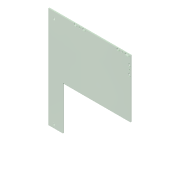
# Autodesk Inventor part: EE PSU TOP
Saved by Autodesk Inventor 2017 (Build 210142000, 142)
## iProperties
Created: 2016-07-27
Part Number: EE PSU TOP
Material: Polycarbonate, Green
Document SubType Name: Modeling
Designer: User
Density: 1.2 g/cm^3
Appearance: Polycarbonate - Clear(2)
Author: User
Autodesk Inventor part; units mm, degrees
ref_plane "YZ Plane" through (0, 0, 0) normal (1, 0, 0) x (0, 1, 0)
ref_plane "XZ Plane" through (0, 0, 0) normal (0, 1, 0) x (-1, 0, 0)
ref_plane "XY Plane" through (0, 0, 0) normal (0, 0, 1) x (1, 0, 0)
sketch "Sketch1" plane through (0, 0, 0) normal (0, 1, 0) x (-1, 0, 0)
  line L0 (55.2995, 771.1017) -> (53.2995, 771.1017)
  line L1 (53.2995, 771.1017) -> (53.2995, 769.1016)
  line L2 (53.2995, 769.1016) -> (53.2995, 481.7779)
  line L3 (53.2995, 481.7779) -> (65.4836, 481.7779)
  line L4 (65.4836, 481.7779) -> (65.4836, 475.7779)
  line L5 (65.4836, 475.7779) -> (70.4836, 475.7779)
  line L6 (70.4836, 475.7779) -> (70.4836, 481.7779)
  line L7 (70.4836, 481.7779) -> (71.2995, 481.7779)
  line L8 (71.2995, 481.7779) -> (71.2995, 623.7779)
  line L9 (71.2995, 623.7779) -> (225.2995, 623.7779)
  line L10 (225.2995, 623.7779) -> (225.2995, 481.7779)
  line L11 (225.2995, 481.7779) -> (234.2995, 481.7779)
  line L12 (234.2995, 481.7779) -> (234.2995, 476.778)
  line L13 (234.2995, 476.778) -> (262.2995, 476.778)
  line L14 (262.2995, 476.778) -> (262.2995, 771.1017)
  line L15 (262.2995, 771.1017) -> (55.2995, 771.1017)
  line L16 (58.3449, 526.6921) -> (58.1851, 527.078)
  line L17 (58.1851, 527.078) -> (57.9308, 527.4094)
  line L18 (57.9308, 527.4094) -> (57.5994, 527.6636)
  line L19 (57.5994, 527.6636) -> (57.2135, 527.8234)
  line L20 (57.2135, 527.8234) -> (56.7994, 527.878)
  line L21 (56.7994, 527.878) -> (56.3853, 527.8234)
  line L22 (56.3853, 527.8234) -> (55.9994, 527.6636)
  line L23 (55.9994, 527.6636) -> (55.668, 527.4093)
  line L24 (55.668, 527.4093) -> (55.4138, 527.0779)
  line L25 (55.4138, 527.0779) -> (55.254, 526.692)
  line L26 (55.254, 526.692) -> (55.1994, 526.2779)
  line L27 (55.1994, 526.2779) -> (55.254, 525.8638)
  line L28 (55.254, 525.8638) -> (55.4138, 525.4779)
  line L29 (55.4138, 525.4779) -> (55.6681, 525.1465)
  line L30 (55.6681, 525.1465) -> (55.9994, 524.8923)
  line L31 (55.9994, 524.8923) -> (56.3853, 524.7325)
  line L32 (56.3853, 524.7325) -> (56.7992, 524.678)
  line L33 (56.7992, 524.678) -> (57.2135, 524.7325)
  line L34 (57.2135, 524.7325) -> (57.5994, 524.8924)
  line L35 (57.5994, 524.8924) -> (57.9308, 525.1466)
  line L36 (57.9308, 525.1466) -> (58.185, 525.478)
  line L37 (58.185, 525.478) -> (58.3449, 525.864)
  line L38 (58.3449, 525.864) -> (58.3994, 526.2781)
  line L39 (58.3994, 526.2781) -> (58.3449, 526.6921)
  line L40 (185.1711, 767.5014) -> (185.0472, 767.8829)
  line L41 (185.0472, 767.8829) -> (184.8323, 768.2215)
  line L42 (184.8323, 768.2215) -> (184.54, 768.496)
  line L43 (184.54, 768.496) -> (184.1885, 768.6893)
  line L44 (184.1885, 768.6893) -> (183.8, 768.7891)
  line L45 (183.8, 768.7891) -> (183.399, 768.7891)
  line L46 (183.399, 768.7891) -> (183.0105, 768.6893)
  line L47 (183.0105, 768.6893) -> (182.659, 768.4961)
  line L48 (182.659, 768.4961) -> (182.3667, 768.2216)
  line L49 (182.3667, 768.2216) -> (182.1518, 767.8829)
  line L50 (182.1518, 767.8829) -> (182.0278, 767.5015)
  line L51 (182.0278, 767.5015) -> (182.0026, 767.1012)
  line L52 (182.0026, 767.1012) -> (182.0778, 766.7072)
  line L53 (182.0778, 766.7072) -> (182.2485, 766.3443)
  line L54 (182.2485, 766.3443) -> (182.5042, 766.0353)
  line L55 (182.5042, 766.0353) -> (182.8287, 765.7996)
  line L56 (182.8287, 765.7996) -> (183.2016, 765.652)
  line L57 (183.2016, 765.652) -> (183.5994, 765.6017)
  line L58 (183.5994, 765.6017) -> (183.9974, 765.652)
  line L59 (183.9974, 765.652) -> (184.3703, 765.7996)
  line L60 (184.3703, 765.7996) -> (184.6947, 766.0353)
  line L61 (184.6947, 766.0353) -> (184.9504, 766.3444)
  line L62 (184.9504, 766.3444) -> (185.1212, 766.7072)
  line L63 (185.1212, 766.7072) -> (185.1963, 767.1012)
  line L64 (185.1963, 767.1012) -> (185.1711, 767.5014)
  line L65 (76.9712, 767.5015) -> (76.8472, 767.8829)
  line L66 (76.8472, 767.8829) -> (76.6323, 768.2216)
  line L67 (76.6323, 768.2216) -> (76.3399, 768.4961)
  line L68 (76.3399, 768.4961) -> (75.9885, 768.6893)
  line L69 (75.9885, 768.6893) -> (75.6, 768.7891)
  line L70 (75.6, 768.7891) -> (75.199, 768.7891)
  line L71 (75.199, 768.7891) -> (74.8105, 768.6893)
  line L72 (74.8105, 768.6893) -> (74.459, 768.4961)
  line L73 (74.459, 768.4961) -> (74.1667, 768.2216)
  line L74 (74.1667, 768.2216) -> (73.9518, 767.8829)
  line L75 (73.9518, 767.8829) -> (73.8278, 767.5015)
  line L76 (73.8278, 767.5015) -> (73.8027, 767.1012)
  line L77 (73.8027, 767.1012) -> (73.8778, 766.7072)
  line L78 (73.8778, 766.7072) -> (74.0486, 766.3444)
  line L79 (74.0486, 766.3444) -> (74.3042, 766.0353)
  line L80 (74.3042, 766.0353) -> (74.6287, 765.7996)
  line L81 (74.6287, 765.7996) -> (75.0016, 765.652)
  line L82 (75.0016, 765.652) -> (75.3995, 765.6017)
  line L83 (75.3995, 765.6017) -> (75.7974, 765.652)
  line L84 (75.7974, 765.652) -> (76.1703, 765.7996)
  line L85 (76.1703, 765.7996) -> (76.4947, 766.0353)
  line L86 (76.4947, 766.0353) -> (76.7504, 766.3444)
  line L87 (76.7504, 766.3444) -> (76.9212, 766.7072)
  line L88 (76.9212, 766.7072) -> (76.9964, 767.1012)
  line L89 (76.9964, 767.1012) -> (76.9712, 767.5015)
  line L90 (250.722, 522.4271) -> (250.4714, 523.032)
  line L91 (250.4714, 523.032) -> (250.0729, 523.5514)
  line L92 (250.0729, 523.5514) -> (249.5534, 523.9499)
  line L93 (249.5534, 523.9499) -> (248.9485, 524.2005)
  line L94 (248.9485, 524.2005) -> (248.2994, 524.286)
  line L95 (248.2994, 524.286) -> (247.6503, 524.2005)
  line L96 (247.6503, 524.2005) -> (247.0454, 523.95)
  line L97 (247.0454, 523.95) -> (246.526, 523.5514)
  line L98 (246.526, 523.5514) -> (246.1275, 523.0319)
  line L99 (246.1275, 523.0319) -> (245.8769, 522.4271)
  line L100 (245.8769, 522.4271) -> (245.7914, 521.778)
  line L101 (245.7914, 521.778) -> (245.8769, 521.1288)
  line L102 (245.8769, 521.1288) -> (246.1275, 520.524)
  line L103 (246.1275, 520.524) -> (246.526, 520.0045)
  line L104 (246.526, 520.0045) -> (247.0455, 519.606)
  line L105 (247.0455, 519.606) -> (247.6504, 519.3555)
  line L106 (247.6504, 519.3555) -> (248.2995, 519.27)
  line L107 (248.2995, 519.27) -> (248.9486, 519.3554)
  line L108 (248.9486, 519.3554) -> (249.5535, 519.606)
  line L109 (249.5535, 519.606) -> (250.0729, 520.0046)
  line L110 (250.0729, 520.0046) -> (250.4714, 520.524)
  line L111 (250.4714, 520.524) -> (250.722, 521.1289)
  line L112 (250.722, 521.1289) -> (250.8075, 521.7779)
  line L113 (250.8075, 521.7779) -> (250.722, 522.4271)
  line L114 (250.7224, 754.4272) -> (250.4718, 755.0321)
  line L115 (250.4718, 755.0321) -> (250.0733, 755.5515)
  line L116 (250.0733, 755.5515) -> (249.5538, 755.95)
  line L117 (249.5538, 755.95) -> (248.9489, 756.2005)
  line L118 (248.9489, 756.2005) -> (248.2998, 756.286)
  line L119 (248.2998, 756.286) -> (247.6507, 756.2006)
  line L120 (247.6507, 756.2006) -> (247.0458, 755.95)
  line L121 (247.0458, 755.95) -> (246.5264, 755.5515)
  line L122 (246.5264, 755.5515) -> (246.1279, 755.032)
  line L123 (246.1279, 755.032) -> (245.8773, 754.4271)
  line L124 (245.8773, 754.4271) -> (245.7918, 753.778)
  line L125 (245.7918, 753.778) -> (245.8773, 753.1288)
  line L126 (245.8773, 753.1288) -> (246.1279, 752.524)
  line L127 (246.1279, 752.524) -> (246.5264, 752.0045)
  line L128 (246.5264, 752.0045) -> (247.0459, 751.606)
  line L129 (247.0459, 751.606) -> (247.6508, 751.3555)
  line L130 (247.6508, 751.3555) -> (248.2999, 751.27)
  line L131 (248.2999, 751.27) -> (248.949, 751.3555)
  line L132 (248.949, 751.3555) -> (249.5539, 751.606)
  line L133 (249.5539, 751.606) -> (250.0737, 752.0049)
  line L134 (250.0737, 752.0049) -> (250.4719, 752.5239)
  line L135 (250.4719, 752.5239) -> (250.7224, 753.1288)
  line L136 (250.7224, 753.1288) -> (250.8079, 753.7777)
  line L137 (250.8079, 753.7777) -> (250.7224, 754.4272)
  line L138 (82.8995, 769.1016) -> (82.8995, 765.5017)
  line L139 (82.8995, 765.5017) -> (89.0995, 765.5017)
  line L140 (89.0995, 765.5017) -> (89.0995, 769.1016)
  line L141 (89.0995, 769.1016) -> (82.8995, 769.1016)
  line L142 (169.8995, 769.1016) -> (169.8995, 765.5017)
  line L143 (169.8995, 765.5017) -> (176.0995, 765.5017)
  line L144 (176.0995, 765.5017) -> (176.0995, 769.1016)
  line L145 (176.0995, 769.1016) -> (169.8995, 769.1016)
  line L146 (191.0995, 769.1016) -> (191.0995, 765.5017)
  line L147 (191.0995, 765.5017) -> (197.2995, 765.5017)
  line L148 (197.2995, 765.5017) -> (197.2995, 769.1016)
  line L149 (197.2995, 769.1016) -> (191.0995, 769.1016)
  line L150 (55.2995, 518.7672) -> (55.2995, 512.5672)
  line L151 (55.2995, 512.5672) -> (58.8995, 512.5672)
  line L152 (58.8995, 512.5672) -> (58.8995, 518.7672)
  line L153 (58.8995, 518.7672) -> (55.2995, 518.7672)
  line L154 (55.2995, 729.278) -> (55.2995, 723.0779)
  line L155 (55.2995, 723.0779) -> (58.8995, 723.0779)
  line L156 (58.8995, 723.0779) -> (58.8995, 729.278)
  line L157 (58.8995, 729.278) -> (55.2995, 729.278)
  line L158 (58.3568, 737.2044) -> (58.197, 737.5902)
  line L159 (58.197, 737.5902) -> (57.9428, 737.9216)
  line L160 (57.9428, 737.9216) -> (57.6114, 738.1758)
  line L161 (57.6114, 738.1758) -> (57.2255, 738.3357)
  line L162 (57.2255, 738.3357) -> (56.8114, 738.3902)
  line L163 (56.8114, 738.3902) -> (56.3972, 738.3357)
  line L164 (56.3972, 738.3357) -> (56.0113, 738.1758)
  line L165 (56.0113, 738.1758) -> (55.68, 737.9216)
  line L166 (55.68, 737.9216) -> (55.4258, 737.5902)
  line L167 (55.4258, 737.5902) -> (55.2659, 737.2043)
  line L168 (55.2659, 737.2043) -> (55.2114, 736.7902)
  line L169 (55.2114, 736.7902) -> (55.2659, 736.3761)
  line L170 (55.2659, 736.3761) -> (55.4257, 735.9902)
  line L171 (55.4257, 735.9902) -> (55.68, 735.6588)
  line L172 (55.68, 735.6588) -> (56.0114, 735.4046)
  line L173 (56.0114, 735.4046) -> (56.3973, 735.2448)
  line L174 (56.3973, 735.2448) -> (56.8114, 735.1902)
  line L175 (56.8114, 735.1902) -> (57.2255, 735.2447)
  line L176 (57.2255, 735.2447) -> (57.6114, 735.4046)
  line L177 (57.6114, 735.4046) -> (57.9427, 735.6588)
  line L178 (57.9427, 735.6588) -> (58.197, 735.9903)
  line L179 (58.197, 735.9903) -> (58.3568, 736.3762)
  line L180 (58.3568, 736.3762) -> (58.4114, 736.7902)
  line L181 (58.4114, 736.7902) -> (58.3568, 737.2044)
  line L182 (58.0995, 769.1016) -> (58.0995, 765.5017)
  line L183 (58.0995, 765.5017) -> (67.8995, 765.5017)
  line L184 (67.8995, 765.5017) -> (67.8995, 769.1016)
  line L185 (67.8995, 769.1016) -> (58.0995, 769.1016)
  line L186 (55.2995, 750.4779) -> (55.2995, 744.2779)
  line L187 (55.2995, 744.2779) -> (58.8995, 744.2779)
  line L188 (58.8995, 744.2779) -> (58.8995, 750.4779)
  line L189 (58.8995, 750.4779) -> (55.2995, 750.4779)
  line L190 (55.2995, 539.9672) -> (55.2995, 533.7672)
  line L191 (55.2995, 533.7672) -> (58.8995, 533.7672)
  line L192 (58.8995, 533.7672) -> (58.8995, 539.9672)
  line L193 (58.8995, 539.9672) -> (55.2995, 539.9672)
  point P0 (0, 0)
  constraints: 388 end point, 97 parallel, 60 perpendicular, 4 collinear
extrude "Extrusion1" add sketch "Sketch1" along normal blind 3
sketch "Sketch2" plane through (0, 3, 0) normal (0, 1, 0) x (1, 0, 0)
  line L0 (-58.0995, -769.1016) -> (-67.8995, -769.1016) projected
  line L1 (-67.8995, -769.1016) -> (-67.8995, -765.5017) projected
  line L2 (-67.8995, -765.5017) -> (-58.0995, -765.5017) projected
  line L3 (-58.0995, -765.5017) -> (-58.0995, -769.1016) projected
  line L4 (-55.2995, -729.278) -> (-58.8995, -729.278) projected
  line L5 (-58.8995, -729.278) -> (-58.8995, -723.0779) projected
  line L6 (-58.8995, -723.0779) -> (-55.2995, -723.0779) projected
  line L7 (-55.2995, -723.0779) -> (-55.2995, -729.278) projected
  line L8 (-55.2995, -518.7672) -> (-58.8995, -518.7672) projected
  line L9 (-58.8995, -518.7672) -> (-58.8995, -512.5672) projected
  line L10 (-58.8995, -512.5672) -> (-55.2995, -512.5672) projected
  line L11 (-55.2995, -512.5672) -> (-55.2995, -518.7672) projected
  line L12 (-191.0995, -769.1016) -> (-197.2995, -769.1016) projected
  line L13 (-197.2995, -769.1016) -> (-197.2995, -765.5017) projected
  line L14 (-197.2995, -765.5017) -> (-191.0995, -765.5017) projected
  line L15 (-191.0995, -765.5017) -> (-191.0995, -769.1016) projected
  line L16 (-55.2995, -539.9672) -> (-58.8995, -539.9672) projected
  line L17 (-58.8995, -539.9672) -> (-58.8995, -533.7672) projected
  line L18 (-58.8995, -533.7672) -> (-55.2995, -533.7672) projected
  line L19 (-55.2995, -533.7672) -> (-55.2995, -539.9672) projected
  line L20 (-55.2995, -750.4779) -> (-58.8995, -750.4779) projected
  line L21 (-58.8995, -750.4779) -> (-58.8995, -744.2779) projected
  line L22 (-58.8995, -744.2779) -> (-55.2995, -744.2779) projected
  line L23 (-55.2995, -744.2779) -> (-55.2995, -750.4779) projected
  line L24 (-169.8995, -769.1016) -> (-176.0995, -769.1016) projected
  line L25 (-176.0995, -769.1016) -> (-176.0995, -765.5017) projected
  line L26 (-176.0995, -765.5017) -> (-169.8995, -765.5017) projected
  line L27 (-169.8995, -765.5017) -> (-169.8995, -769.1016) projected
  line L28 (-82.8995, -769.1016) -> (-89.0995, -769.1016) projected
  line L29 (-89.0995, -769.1016) -> (-89.0995, -765.5017) projected
  line L30 (-89.0995, -765.5017) -> (-82.8995, -765.5017) projected
  line L31 (-82.8995, -765.5017) -> (-82.8995, -769.1016) projected
  line L32 (-250.7224, -754.4272) -> (-250.8079, -753.7777) projected
  line L33 (-250.8079, -753.7777) -> (-250.7224, -753.1288) projected
  line L34 (-250.7224, -753.1288) -> (-250.4719, -752.5239) projected
  line L35 (-250.4719, -752.5239) -> (-250.0737, -752.0049) projected
  line L36 (-250.0737, -752.0049) -> (-249.5539, -751.606) projected
  line L37 (-249.5539, -751.606) -> (-248.949, -751.3555) projected
  line L38 (-248.949, -751.3555) -> (-248.2999, -751.27) projected
  line L39 (-248.2999, -751.27) -> (-247.6508, -751.3555) projected
  line L40 (-247.6508, -751.3555) -> (-247.0459, -751.606) projected
  line L41 (-247.0459, -751.606) -> (-246.5264, -752.0045) projected
  line L42 (-246.5264, -752.0045) -> (-246.1279, -752.524) projected
  line L43 (-246.1279, -752.524) -> (-245.8773, -753.1288) projected
  line L44 (-245.8773, -753.1288) -> (-245.7918, -753.778) projected
  line L45 (-245.7918, -753.778) -> (-245.8773, -754.4271) projected
  line L46 (-245.8773, -754.4271) -> (-246.1279, -755.032) projected
  line L47 (-246.1279, -755.032) -> (-246.5264, -755.5515) projected
  line L48 (-246.5264, -755.5515) -> (-247.0458, -755.95) projected
  line L49 (-247.0458, -755.95) -> (-247.6507, -756.2006) projected
  line L50 (-247.6507, -756.2006) -> (-248.2998, -756.286) projected
  line L51 (-248.2998, -756.286) -> (-248.9489, -756.2005) projected
  line L52 (-248.9489, -756.2005) -> (-249.5538, -755.95) projected
  line L53 (-249.5538, -755.95) -> (-250.0733, -755.5515) projected
  line L54 (-250.0733, -755.5515) -> (-250.4718, -755.0321) projected
  line L55 (-250.4718, -755.0321) -> (-250.7224, -754.4272) projected
  line L56 (-250.722, -522.4271) -> (-250.8075, -521.7779) projected
  line L57 (-250.8075, -521.7779) -> (-250.722, -521.1289) projected
  line L58 (-250.722, -521.1289) -> (-250.4714, -520.524) projected
  line L59 (-250.4714, -520.524) -> (-250.0729, -520.0046) projected
  line L60 (-250.0729, -520.0046) -> (-249.5535, -519.606) projected
  line L61 (-249.5535, -519.606) -> (-248.9486, -519.3554) projected
  line L62 (-248.9486, -519.3554) -> (-248.2995, -519.27) projected
  line L63 (-248.2995, -519.27) -> (-247.6504, -519.3555) projected
  line L64 (-247.6504, -519.3555) -> (-247.0455, -519.606) projected
  line L65 (-247.0455, -519.606) -> (-246.526, -520.0045) projected
  line L66 (-246.526, -520.0045) -> (-246.1275, -520.524) projected
  line L67 (-246.1275, -520.524) -> (-245.8769, -521.1288) projected
  line L68 (-245.8769, -521.1288) -> (-245.7914, -521.778) projected
  line L69 (-245.7914, -521.778) -> (-245.8769, -522.4271) projected
  line L70 (-245.8769, -522.4271) -> (-246.1275, -523.0319) projected
  line L71 (-246.1275, -523.0319) -> (-246.526, -523.5514) projected
  line L72 (-246.526, -523.5514) -> (-247.0454, -523.95) projected
  line L73 (-247.0454, -523.95) -> (-247.6503, -524.2005) projected
  line L74 (-247.6503, -524.2005) -> (-248.2994, -524.286) projected
  line L75 (-248.2994, -524.286) -> (-248.9485, -524.2005) projected
  line L76 (-248.9485, -524.2005) -> (-249.5534, -523.9499) projected
  line L77 (-249.5534, -523.9499) -> (-250.0729, -523.5514) projected
  line L78 (-250.0729, -523.5514) -> (-250.4714, -523.032) projected
  line L79 (-250.4714, -523.032) -> (-250.722, -522.4271) projected
  line L80 (-76.9712, -767.5015) -> (-76.9964, -767.1012) projected
  line L81 (-76.9964, -767.1012) -> (-76.9212, -766.7072) projected
  line L82 (-76.9212, -766.7072) -> (-76.7504, -766.3444) projected
  line L83 (-76.7504, -766.3444) -> (-76.4947, -766.0353) projected
  line L84 (-76.4947, -766.0353) -> (-76.1703, -765.7996) projected
  line L85 (-76.1703, -765.7996) -> (-75.7974, -765.652) projected
  line L86 (-75.7974, -765.652) -> (-75.3995, -765.6017) projected
  line L87 (-75.3995, -765.6017) -> (-75.0016, -765.652) projected
  line L88 (-75.0016, -765.652) -> (-74.6287, -765.7996) projected
  line L89 (-74.6287, -765.7996) -> (-74.3042, -766.0353) projected
  line L90 (-74.3042, -766.0353) -> (-74.0486, -766.3444) projected
  line L91 (-74.0486, -766.3444) -> (-73.8778, -766.7072) projected
  line L92 (-73.8778, -766.7072) -> (-73.8027, -767.1012) projected
  line L93 (-73.8027, -767.1012) -> (-73.8278, -767.5015) projected
  line L94 (-73.8278, -767.5015) -> (-73.9518, -767.8829) projected
  line L95 (-73.9518, -767.8829) -> (-74.1667, -768.2216) projected
  line L96 (-74.1667, -768.2216) -> (-74.459, -768.4961) projected
  line L97 (-74.459, -768.4961) -> (-74.8105, -768.6893) projected
  line L98 (-74.8105, -768.6893) -> (-75.199, -768.7891) projected
  line L99 (-75.199, -768.7891) -> (-75.6, -768.7891) projected
  line L100 (-75.6, -768.7891) -> (-75.9885, -768.6893) projected
  line L101 (-75.9885, -768.6893) -> (-76.3399, -768.4961) projected
  line L102 (-76.3399, -768.4961) -> (-76.6323, -768.2216) projected
  line L103 (-76.6323, -768.2216) -> (-76.8472, -767.8829) projected
  line L104 (-76.8472, -767.8829) -> (-76.9712, -767.5015) projected
  line L105 (-185.1711, -767.5014) -> (-185.1963, -767.1012) projected
  line L106 (-185.1963, -767.1012) -> (-185.1212, -766.7072) projected
  line L107 (-185.1212, -766.7072) -> (-184.9504, -766.3444) projected
  line L108 (-184.9504, -766.3444) -> (-184.6947, -766.0353) projected
  line L109 (-184.6947, -766.0353) -> (-184.3703, -765.7996) projected
  line L110 (-184.3703, -765.7996) -> (-183.9974, -765.652) projected
  line L111 (-183.9974, -765.652) -> (-183.5994, -765.6017) projected
  line L112 (-183.5994, -765.6017) -> (-183.2016, -765.652) projected
  line L113 (-183.2016, -765.652) -> (-182.8287, -765.7996) projected
  line L114 (-182.8287, -765.7996) -> (-182.5042, -766.0353) projected
  line L115 (-182.5042, -766.0353) -> (-182.2485, -766.3443) projected
  line L116 (-182.2485, -766.3443) -> (-182.0778, -766.7072) projected
  line L117 (-182.0778, -766.7072) -> (-182.0026, -767.1012) projected
  line L118 (-182.0026, -767.1012) -> (-182.0278, -767.5015) projected
  line L119 (-182.0278, -767.5015) -> (-182.1518, -767.8829) projected
  line L120 (-182.1518, -767.8829) -> (-182.3667, -768.2216) projected
  line L121 (-182.3667, -768.2216) -> (-182.659, -768.4961) projected
  line L122 (-182.659, -768.4961) -> (-183.0105, -768.6893) projected
  line L123 (-183.0105, -768.6893) -> (-183.399, -768.7891) projected
  line L124 (-183.399, -768.7891) -> (-183.8, -768.7891) projected
  line L125 (-183.8, -768.7891) -> (-184.1885, -768.6893) projected
  line L126 (-184.1885, -768.6893) -> (-184.54, -768.496) projected
  line L127 (-184.54, -768.496) -> (-184.8323, -768.2215) projected
  line L128 (-184.8323, -768.2215) -> (-185.0472, -767.8829) projected
  line L129 (-185.0472, -767.8829) -> (-185.1711, -767.5014) projected
  line L130 (-58.3568, -737.2044) -> (-58.4114, -736.7902) projected
  line L131 (-58.4114, -736.7902) -> (-58.3568, -736.3762) projected
  line L132 (-58.3568, -736.3762) -> (-58.197, -735.9903) projected
  line L133 (-58.197, -735.9903) -> (-57.9427, -735.6588) projected
  line L134 (-57.9427, -735.6588) -> (-57.6114, -735.4046) projected
  line L135 (-57.6114, -735.4046) -> (-57.2255, -735.2447) projected
  line L136 (-57.2255, -735.2447) -> (-56.8114, -735.1902) projected
  line L137 (-56.8114, -735.1902) -> (-56.3973, -735.2448) projected
  line L138 (-56.3973, -735.2448) -> (-56.0114, -735.4046) projected
  line L139 (-56.0114, -735.4046) -> (-55.68, -735.6588) projected
  line L140 (-55.68, -735.6588) -> (-55.4257, -735.9902) projected
  line L141 (-55.4257, -735.9902) -> (-55.2659, -736.3761) projected
  line L142 (-55.2659, -736.3761) -> (-55.2114, -736.7902) projected
  line L143 (-55.2114, -736.7902) -> (-55.2659, -737.2043) projected
  line L144 (-55.2659, -737.2043) -> (-55.4258, -737.5902) projected
  line L145 (-55.4258, -737.5902) -> (-55.68, -737.9216) projected
  line L146 (-55.68, -737.9216) -> (-56.0113, -738.1758) projected
  line L147 (-56.0113, -738.1758) -> (-56.3972, -738.3357) projected
  line L148 (-56.3972, -738.3357) -> (-56.8114, -738.3902) projected
  line L149 (-56.8114, -738.3902) -> (-57.2255, -738.3357) projected
  line L150 (-57.2255, -738.3357) -> (-57.6114, -738.1758) projected
  line L151 (-57.6114, -738.1758) -> (-57.9428, -737.9216) projected
  line L152 (-57.9428, -737.9216) -> (-58.197, -737.5902) projected
  line L153 (-58.197, -737.5902) -> (-58.3568, -737.2044) projected
  line L154 (-58.3449, -526.6921) -> (-58.3994, -526.2781) projected
  line L155 (-58.3994, -526.2781) -> (-58.3449, -525.864) projected
  line L156 (-58.3449, -525.864) -> (-58.185, -525.478) projected
  line L157 (-58.185, -525.478) -> (-57.9308, -525.1466) projected
  line L158 (-57.9308, -525.1466) -> (-57.5994, -524.8924) projected
  line L159 (-57.5994, -524.8924) -> (-57.2135, -524.7325) projected
  line L160 (-57.2135, -524.7325) -> (-56.7992, -524.678) projected
  line L161 (-56.7992, -524.678) -> (-56.3853, -524.7325) projected
  line L162 (-56.3853, -524.7325) -> (-55.9994, -524.8923) projected
  line L163 (-55.9994, -524.8923) -> (-55.6681, -525.1465) projected
  line L164 (-55.6681, -525.1465) -> (-55.4138, -525.4779) projected
  line L165 (-55.4138, -525.4779) -> (-55.254, -525.8638) projected
  line L166 (-55.254, -525.8638) -> (-55.1994, -526.2779) projected
  line L167 (-55.1994, -526.2779) -> (-55.254, -526.692) projected
  line L168 (-55.254, -526.692) -> (-55.4138, -527.0779) projected
  line L169 (-55.4138, -527.0779) -> (-55.668, -527.4093) projected
  line L170 (-55.668, -527.4093) -> (-55.9994, -527.6636) projected
  line L171 (-55.9994, -527.6636) -> (-56.3853, -527.8234) projected
  line L172 (-56.3853, -527.8234) -> (-56.7994, -527.878) projected
  line L173 (-56.7994, -527.878) -> (-57.2135, -527.8234) projected
  line L174 (-57.2135, -527.8234) -> (-57.5994, -527.6636) projected
  line L175 (-57.5994, -527.6636) -> (-57.9308, -527.4094) projected
  line L176 (-57.9308, -527.4094) -> (-58.1851, -527.078) projected
  line L177 (-58.1851, -527.078) -> (-58.3449, -526.6921) projected
  line L178 (-262.2995, -771.1017) -> (-53.2995, -771.1017) projected
  line L179 (-53.2995, -771.1017) -> (-53.2995, -481.7779) projected
  line L180 (-53.2995, -481.7779) -> (-65.4836, -481.7779) projected
  line L181 (-65.4836, -481.7779) -> (-65.4836, -475.7779) projected
  line L182 (-65.4836, -475.7779) -> (-70.4836, -475.7779) projected
  line L183 (-70.4836, -475.7779) -> (-70.4836, -481.7779) projected
  line L184 (-70.4836, -481.7779) -> (-71.2995, -481.7779) projected
  line L185 (-71.2995, -481.7779) -> (-71.2995, -623.7779) projected
  line L186 (-71.2995, -623.7779) -> (-225.2995, -623.7779) projected
  line L187 (-225.2995, -623.7779) -> (-225.2995, -481.7779) projected
  line L188 (-225.2995, -481.7779) -> (-234.2995, -481.7779) projected
  line L189 (-234.2995, -481.7779) -> (-234.2995, -476.778) projected
  line L190 (-234.2995, -476.778) -> (-262.2995, -476.778) projected
  line L191 (-262.2995, -476.778) -> (-262.2995, -771.1017) projected
  circle A0 centre (-75.3995, -767.2017) radius 1.5874
  circle A1 centre (-183.5995, -767.2017) radius 1.5874
  circle A2 centre (-56.8114, -736.7902) radius 1.5863
  circle A3 centre (-56.7995, -526.278) radius 1.5862
  point P0 (0, 0)
  constraints: 12 tangent, 4 centre point
hole "Hole1" at (-56.7995, 3, 526.278) at (-56.8114, 3, 736.7902) at (-75.3995, 3, 767.2017) at (-183.5995, 3, 767.2017) direction (0, -1, 0) diameter 3.2 end through all
sketch "Sketch5" plane through (0, 3, 0) normal (0, 1, 0) x (1, 0, 0)
  line L0 (-247.6507, -756.2006) -> (-247.0458, -755.95) projected
  line L1 (-250.0733, -755.5515) -> (-249.5538, -755.95) projected
  line L2 (-248.949, -751.3555) -> (-248.2999, -751.27) projected
  line L3 (-248.9486, -519.3554) -> (-248.2995, -519.27) projected
  line L4 (-249.5534, -523.9499) -> (-250.0729, -523.5514) projected
  line L5 (-246.526, -523.5514) -> (-247.0454, -523.95) projected
  circle A0 centre (-248.2998, -753.778) radius 2.4866
  circle A1 centre (-248.2994, -521.778) radius 2.4866
  point P0 (0, 0)
  constraints: 6 tangent, 2 centre point
hole "Hole2" at (-248.2998, 3, 753.778) at (-248.2994, 3, 521.778) direction (0, -1, 0) diameter 5.2 end through all
sketch "Sketch6" plane through (0, 3, 0) normal (0, 1, 0) x (1, 0, 0)
  line L0 (-71.2995, -481.7779) -> (-71.2995, -623.7779) projected
  line L1 (-71.2995, -481.7779) -> (-53.2995, -481.7779)
  line L2 (-53.2995, -481.7779) -> (-53.2995, -455.7908)
  line L3 (-53.2995, -455.7908) -> (-71.2995, -455.7908)
  line L4 (-71.2995, -455.7908) -> (-71.2995, -481.7779)
  point P0 (0, 0)
  constraints: 8 end point, 2 parallel, 1 horizontal, 1 perpendicular
extrude "Extrusion2" add sketch "Sketch6" against normal blind 3
sketch "Sketch7" plane through (0, 3, 0) normal (0, 1, 0) x (1, 0, 0)
  circle A0 centre (-62.3818, -460.5756) radius 2.6
  point P0 (0, 0)
  point P1 (-187.2996, -460.5756)
  dimension "d18" = 5.2
  constraints: 1 centre point, 4 other
  measures "d18" diameter of A0
extrude "Extrusion3" cut sketch "Sketch7" against normal through all
sketch "Sketch8" plane through (0, 3, 0) normal (0, 1, 0) x (1, 0, 0)
  line L0 (-221.4165, -513.2612) -> (-270.0696, -513.2612)
  line L1 (-270.0696, -513.2612) -> (-270.0696, -464.0531)
  line L2 (-270.0696, -464.0531) -> (-221.4165, -464.0531)
  line L3 (-221.4165, -464.0531) -> (-221.4165, -513.2612)
  point P0 (0, 0)
  point P1 (-236.6995, -510.7779)
  constraints: 8 end point, 2 parallel, 1 horizontal, 1 perpendicular, 1 other
extrude "Extrusion4" cut sketch "Sketch8" against normal blind 3
sketch "Sketch9" plane through (0, 3, 0) normal (0, 1, 0) x (1, 0, 0)
  line L0 (-71.2995, -623.7779) -> (-25.9421, -623.7779)
  line L1 (-25.9421, -623.7779) -> (-25.9421, -372.5945)
  line L2 (-25.9421, -372.5945) -> (-71.2995, -372.5945)
  line L3 (-71.2995, -372.5945) -> (-71.2995, -623.7779)
  point P0 (0, 0)
  constraints: 8 end point, 2 parallel, 1 horizontal, 1 perpendicular
extrude "Extrusion5" cut sketch "Sketch9" against normal through all
body "Solid1"
